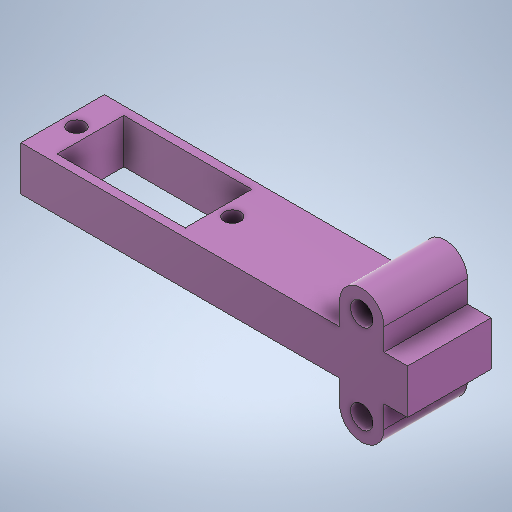
# Autodesk Inventor part: servo_holder
Saved by Autodesk Inventor 2025.1 (Build 291241000, 241)
## iProperties
Created: 2025-02-14
Part Number: servo_holder
Material: Generic
Document SubType Name: Modeling
Designer: m_kni
Density: 1 g/cm^3
Appearance: Default
Author: m_kni
Autodesk Inventor part; units mm, degrees
ref_plane "YZ Plane" through (0, 0, 0) normal (1, 0, 0) x (0, 1, 0)
ref_plane "XZ Plane" through (0, 0, 0) normal (0, 1, 0) x (-1, 0, 0)
ref_plane "XY Plane" through (0, 0, 0) normal (0, 0, 1) x (1, 0, 0)
sketch "Sketch1" plane through (0, 0, 0) normal (0, 1, 0) x (-1, 0, 0)
  line L0 (-25.5949, 6.1189) -> (0.4051, 6.1189)
  line L1 (-25.5949, 6.1189) -> (0.4051, 6.1189)
  line L2 (0.4051, 6.1189) -> (0.4051, -8.8811)
  line L3 (0.4051, -8.8811) -> (-25.5949, -8.8811)
  line L4 (-25.5949, -8.8811) -> (-25.5949, 6.1189)
  line L5 (0.4051, -8.8811) -> (27.4051, -8.8811)
  line L6 (27.4051, -8.8811) -> (27.4051, 6.1189)
  line L7 (27.4051, 6.1189) -> (0.4051, 6.1189)
  line L8 (0.4051, 6.1189) -> (0.4051, -8.8811)
  line L9 (22.4051, -1.3811) -> (22.4051, -7.3811)
  line L10 (22.4051, -7.3811) -> (22.4051, 4.6189)
  line L11 (22.4051, 4.6189) -> (-0.5949, 4.6189)
  line L12 (-0.5949, 4.6189) -> (-0.5949, -7.3811)
  line L13 (-0.5949, -7.3811) -> (22.4051, -7.3811)
  line L14 (22.4051, -1.3811) -> (27.4051, -1.3811)
  circle A0 centre (24.9051, -1.3811) radius 1.5
  line L15 (-0.5949, -1.3811) -> (-5.5949, -1.3811)
  circle A1 centre (-3.0949, -1.3811) radius 1.5
  point P0 (0, 0)
  dimension "d0" = 15
  dimension "d1" = 27
  dimension "d2" = 5
  dimension "d3" = 6
  dimension "d4" = 12
  dimension "d5" = 23
  dimension "d6" = 5
  dimension "d7" = 3
  dimension "d8" = 5
  dimension "d9" = 3
  constraints: 32 end point, 5 parallel, 4 midpoint, 4 perpendicular, 3 horizontal, 2 centre point, 2 point on line, 1 vertical
  measures "d0" distance of L1.end L3.start
  measures "d1" distance of L8.start L7.start
  measures "d2" distance from line of L14.start L6
  measures "d3" distance of L14.start L13.end
  measures "d4" distance of L13.end L11.start
  measures "d5" distance of L11.start L12.start
  measures "d6" distance of L14.start L14.end
  measures "d7" diameter of A0
  measures "d8" distance of L15.start L15.end
  measures "d9" diameter of A1
extrude "Extrusion1" add sketch "Sketch1" along normal blind 8 contours L0 L2 L11 L12 L13 L3 L4 | L7 L6 L14 A0 L10 L11 L2 | L2 L13 L9 L14 A0 L6 L5
sketch "Sketch4" plane through (-27.4051, 0, 6.1189) normal (0, 0, 1) x (1, 0, 0)
  line L0 (53, 8) -> (69.5, 8)
  line L1 (69.5, 8) -> (69.5, 0)
  line L2 (69.5, 0) -> (53, 0)
  line L3 (53, 0) -> (53, 8)
  point P0 (27.4051, 0)
  dimension "d24" = 16.5
  constraints: 8 end point, 2 parallel, 1 horizontal, 1 perpendicular
  measures "d24" distance of L1.end L2.end
extrude "Extrusion3" add sketch "Sketch4" against normal up to surface (15 mm away)
sketch "Sketch5" plane through (-27.4051, 0, 6.1189) normal (0, 0, 1) x (1, 0, 0)
  line L0 (69.5, 0) -> (69.5, 8) projected
  line L1 (69.5, 0) -> (69.5, 8) projected
  line L2 (61.25, 4) -> (61.25, 12)
  line L3 (61.25, 12) -> (61.25, -4)
  circle A0 centre (61.25, 12) radius 2.025
  circle A1 centre (61.25, -4) radius 2.025
  circle A2 centre (61.25, 12) radius 4
  circle A3 centre (61.25, -4) radius 4
  line L4 (57.25, 12) -> (57.25, -4)
  line L5 (65.25, -4) -> (65.25, 12)
  point P0 (27.4051, 0)
  point P1 (69.5, 4)
  point P2 (69.5, 4)
  dimension "d27" = 8.25
  dimension "d28" = 8
  dimension "d29" = 16
  dimension "d30" = 4.05
  dimension "d31" = 4.05
  dimension "d32" = 8
  dimension "d33" = 8
  constraints: 8 end point, 4 centre point, 4 coincident, 4 point on circle, 2 midpoint, 2 vertical, 1 point on line, 1 tangent
  measures "d27" distance of point (69.5, 4) L2.start
  measures "d28" distance of L2.start L2.end
  measures "d29" distance of L2.end L3.end
  measures "d30" diameter of A0
  measures "d31" diameter of A1
  measures "d32" diameter of A2
  measures "d33" diameter of A3
extrude "Extrusion4" add sketch "Sketch5" against normal up to surface (15 mm away)
body "Solid1"
